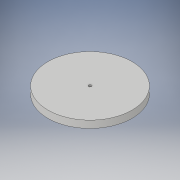
# Autodesk Inventor part: Wheel
Saved by Autodesk Inventor 2019.2 (Build 232265000, 265)
## iProperties
Created: 2019-05-20
Part Number: Wheel
Material: Generic
Document SubType Name: Modeling
Designer: Johansson
Density: 1 g/cm^3
Appearance: Default
Author: Johansson
Autodesk Inventor part; units mm, degrees
ref_plane "YZ Plane" through (0, 0, 0) normal (1, 0, 0) x (0, 1, 0)
ref_plane "XZ Plane" through (0, 0, 0) normal (0, 1, 0) x (-1, 0, 0)
ref_plane "XY Plane" through (0, 0, 0) normal (0, 0, 1) x (1, 0, 0)
sketch "Sketch1" plane through (0, 0, 0) normal (0, 1, 0) x (-1, 0, 0)
  circle A0 centre (0, 0) radius 117.5
  circle A1 centre (0, 0) radius 4
  dimension "d0" = 235
  dimension "d1" = 8
  constraints: 2 centre point, 2 coincident
  measures "d0" diameter of A0
  measures "d1" diameter of A1
extrude "Extrusion1" add sketch "Sketch1" along normal blind 20
equation "\"d0\" = D_Wheel"
equation "\"d1\" = D_Shaft_BLDC"
equation "\"DO_BLDC\" = 63"
equation "\"WO_BLDC\" = 64"
equation "\"D_Shaft_BLDC\" = 8"
equation "\"D_Hole_BLDC\" = 45.5"
equation "\"D_Wheel\" = 235"
equation "\"W_Wall\" = 8"
body "Solid1"
